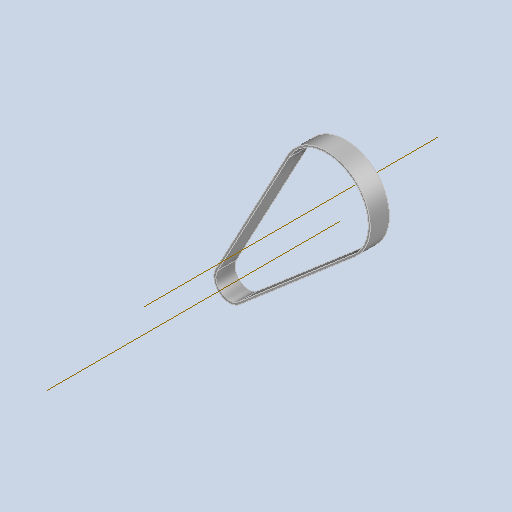
# Autodesk Inventor part: 동기식 벨트
Saved by Autodesk Inventor 2025.3 (Build 293356030, 356C)
## iProperties
Created: 2025-09-07
Part Number: 동기식 벨트
Material: Rubber
Document SubType Name: Modeling
Designer: MSI
Density: 1 g/cm^3
Appearance: Rubber - Black - Version 1.1
CustomPartVersion: 1
Author: MSI
Autodesk Inventor part; units mm, degrees
sketch "스케치 경로" plane through (0, 0, 0) normal (0, 0, 1) x (1, 0, 0)
  arc A0 (-108.7273, -119.8287) -> (-87.0297, -137.232) centre (-96.25, -126.5) ccw
  arc A1 (27.661, -38.696) -> (-37.432, 13.514) centre (0, -6.5) ccw
  line L0 (27.661, -38.696) -> (-87.0297, -137.232)
  line L1 (-108.7273, -119.8287) -> (-37.432, 13.514)
  constraints: 4 end point, 4 point on circle, 2 centre point
ref_plane "횡단면 평면" through (-87.0297, -137.232, 0) normal (0.7585, 0.6517, 0) x (0, 0, 1)
ref_plane "작업 평면2" through (-96.25, -126.5, 0) normal (-1, 0, 0) x (0, 0, 1)
ref_plane "작업 평면3" through (0, -6.5, 0) normal (-0.5479, -0.8365, 0) x (0, 0, 1)
sketch "횡단면" plane through (-87.0297, -137.232, 0) normal (0.7585, 0.6517, 0) x (0, 0, 1)
  line L0 (-9.525, 1.3462) -> (9.525, 1.3462)
  line L1 (9.525, 1.3462) -> (9.525, -0.6858)
  line L2 (9.525, -0.6858) -> (-9.525, -0.6858)
  line L3 (-9.525, -0.6858) -> (-9.525, 1.3462)
  line L4 (-9.525, 0) -> (9.525, 0) construction
  point P0 (0, 0)
  point P1 (0, 0)
  dimension "d0" = 19.05
  dimension "d4" = 0.6858
  dimension "d5" = 1.3462
  constraints: 10 end point, 2 parallel, 2 point on line, 1 coincident, 1 horizontal, 1 midpoint, 1 perpendicular, 1 other
  measures "d0" distance between parallel lines of L1 L3
  measures "d4" distance between parallel lines of L2 L4
  measures "d5" distance between parallel lines of L4 L0
sweep "벨트" add profiles "횡단면" path "스케치 경로"
equation "\"d0\" = da_B"
equation "\"d4\" = da_a"
equation "\"d5\" = da_a2"
equation "\"da_B\" = 19.05"
equation "\"da_pb\" = 12.7"
equation "\"da_L\" = 490.68285"
equation "\"da_a\" = 0.6858"
equation "\"da_S\" = 6.1214"
equation "\"da_Beta\" = 20deg"
equation "\"da_Ht\" = 2.286"
equation "\"da_H\" = 4.318"
equation "\"da_a2\" = 1.3462"
body "Solid1"
